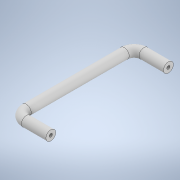
# Autodesk Inventor part: Blechgriff
Saved by Autodesk Inventor 2021.3 (Build 253353000, 353)
## iProperties
Created: 2021-10-19
Part Number: Blechgriff
Material: Generisch
Document SubType Name: Modeling
Designer: bhelg
Density: 1 g/cm^3
Appearance: Vorgabe
Author: bhelg
Autodesk Inventor part; units mm, degrees
ref_plane "YZ Plane" through (0, 0, 0) normal (1, 0, 0) x (0, 1, 0)
ref_plane "XZ Plane" through (0, 0, 0) normal (0, 1, 0) x (-1, 0, 0)
ref_plane "XY Plane" through (0, 0, 0) normal (0, 0, 1) x (1, 0, 0)
sketch "Skizze1" plane through (0, 0, 0) normal (0, 1, 0) x (-1, 0, 0)
  line L0 (0, 0) -> (25, 0)
  line L1 (35, -10) -> (35, -110)
  line L2 (25, -120) -> (0, -120)
  arc A0 (35, -10) -> (25, 0) centre (25, -10) ccw
  arc A1 (25, -120) -> (35, -110) centre (25, -110) ccw
  point P0 (35, 0)
  point P1 (35, -120)
  dimension "d0" = 35
  dimension "d1" = 120
  dimension "d2" = 10
  constraints: 6 end point, 4 point on circle, 4 point on line, 4 tangent, 2 centre point, 2 perpendicular, 1 equal radius, 1 horizontal
  measures "d0" distance of L0.start point (35, 0)
  measures "d1" distance of point (35, 0) point (35, -120)
  measures "d2" radius of A0
sketch "Skizze2" plane through (0, 0, 0) normal (1, 0, 0) x (0, 1, 0)
  circle A0 centre (0, 0) radius 5
  dimension "d3" = 10
  constraints: 1 centre point, 1 coincident
  measures "d3" diameter of A0
sweep "Sweeping1" add profiles "Skizze2" path "Skizze1"
sketch "Skizze3" plane through (0, 0, 0) normal (1, 0, 0) x (0, 0, -1)
  circle A0 centre (0, 0) radius 5 projected
  point P0 (120, 0)
  constraints: 1 coincident
hole "Bohrung1" at (0, 0, 0) at (0, 0, -120) direction (-1, 0, 0) diameter 3.242 depth 11.8 tip angle 118
